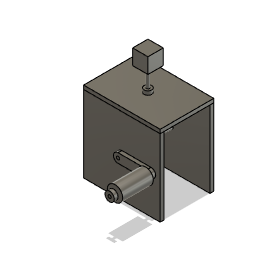
12. カム機構 (Autodesk Fusion 360 design; units mm, degrees)
description: Spur Gear; Module: 2.000000; Num Teeth: 18; Pressure Angle: 20.000000; Backlash: 0.00 mm
description: Spur Gear; Module: 2.000000; Num Teeth: 12; Pressure Angle: 20.000000; Backlash: 0.00 mm
Autodesk Fusion 360 part; units mm, degrees
sketch "スケッチ2" plane through (0, 0, 0) normal (0, 0, 1) x (1, 0, 0)
  line L0 (-25, 0) -> (25, 0)
  line L1 (25, 0) -> (25, 50)
  line L2 (25, 50) -> (-25, 50)
  line L3 (-25, 50) -> (-25, 0)
  circle A0 centre (0, 25) radius 1
  line L4 (3, 57) -> (22, 57)
  arc A1 (22, 57) -> (22, 63) centre (22, 60) ccw
  line L5 (22, 63) -> (3, 63)
  arc A2 (3, 63) -> (3, 57) centre (3, 60) ccw
  line L6 (0, 60) -> (25, 60) construction
  circle A3 centre (3, 60) radius 1
  circle A4 centre (22, 60) radius 1
  circle A5 centre (-15, 60) radius 3
  circle A6 centre (-15, 60) radius 1
  circle A7 centre (-35, 60) radius 5
  circle A8 centre (-35, 60) radius 1.25
  dimension "d1" = 2
  dimension "d16" = 2
  dimension "d21" = 2.5
  constraint horizontal L0
  constraint vertical L1
  constraint horizontal L2
  constraint vertical L3
  constraint tangent L4 A1
  constraint tangent A1 L5
  constraint parallel L4 L5
  constraint tangent L5 A2
  constraint tangent L4 A2
  constraint midpoint A2 L6.start
  constraint midpoint A1 L6.end
  constraint horizontal L6
  constraint concentric A2 A3
  constraint concentric A1 A4
  constraint concentric A5 A6
  constraint concentric A7 A8
  measures "d1" diameter of A0
  measures "d16" diameter of A3
  measures "d21" diameter of A8
extrude "押し出し1" add sketch "スケッチ2" along normal blind 2.5 contours L0 L1 L2 L3 makes body 1
cylinder "円柱プリミティブ1" add diameter 2 height 37.5 placed x (1, 0, 0) y (0, 1, 0) z (0, 0, 1) at (50, 0, 0) separate body makes body 2
extrude "押し出し2" add sketch "スケッチ2" along normal blind 2.5 separate body contours L4 A1 L5 A2 makes body 3
extrude "押し出し3" add sketch "スケッチ2" along normal blind 2.5 separate body contours A5 makes body 4
sketch "スケッチ5" plane through (0, 0, 0) normal (0, 1, 0) x (1, 0, 0)
extrude "押し出し4" add sketch "スケッチ2" along normal blind 20 separate body contours A7 makes body 5
cylinder "円柱プリミティブ2" add diameter 2 height 27 placed x (1, 0, 0) y (0, 1, 0) z (0, 0, 1) at (-25, 60, 0) separate body makes body 6
copy_body "ボディ -> コンポーネント1" bodies 1 removing the originals makes body 7 in component "土台"
copy_body "ボディ -> コンポーネント2" bodies 2 removing the originals makes body 8 in component "軸1"
copy_body "ボディ -> コンポーネント3" bodies 3 removing the originals makes body 9 in component "レバー"
copy_body "ボディ -> コンポーネント4" bodies 4 removing the originals makes body 10 in component "止め輪1"
copy_body "ボディ -> コンポーネント5" bodies 5 removing the originals makes body 11 in component "ハンドル"
copy_body "ボディ -> コンポーネント6" bodies 6 removing the originals makes body 12 in component "軸2"
sketch "スケッチ7" plane through (0, 0, 0) normal (0, 0, 1) x (1, 0, 0)
  line L0 (30, 15) -> (80, 15)
  line L1 (80, 15) -> (80, 50)
  line L2 (80, 50) -> (30, 50)
  line L3 (30, 50) -> (30, 15)
  circle A0 centre (55, 33) radius 1
  circle A1 centre (90, 0) radius 1
  circle A2 centre (100, 0) radius 2.5
  circle A3 centre (100, 0) radius 1
  constraint horizontal L0
  constraint vertical L1
  constraint horizontal L2
  constraint vertical L3
  constraint concentric A2 A3
extrude "押し出し1'" add sketch "スケッチ7" along normal blind 2.5 separate body contours L0 L1 L2 L3 makes body 13 in component "天板"
extrude "押し出し1''" add sketch "スケッチ7" along normal blind 30 separate body contours A1 makes body 14 in component "軸3"
extrude "押し出し1'''" add sketch "スケッチ7" along normal blind 2.5 separate body contours A2 makes body 15 in component "止め輪2"
box "直方体プリミティブ1" add length 10 width 10 height 10 placed x (0, -1, 0) y (1, 0, 0) z (0, 0, 1) at (90, 20, 0) separate body makes body 16 in component "キューブ"
cylinder "円柱プリミティブ1'" cut diameter 2 height -5 placed x (1, 0, 0) y (0, 1, 0) z (0, 0, 1) at (95, 15, 10) bodies 16 in component "キューブ"
extrude "押し出し1''''" add sketch "スケッチ7" along normal blind 2.5 separate body contours A2 makes body 17 in component "止め輪2 (1)"
copy_body "ボディのコピーと貼り付け1" bodies 7 makes body 18 in component "土台"
move_body "移動1" bodies 18 to x (1, 0, 0) y (0, 1, 0) z (0, 0, 1) at (0, 0, -32.5) in component "土台"
component "止め輪1" placed x (1, 0, 0) y (0, 1, 0) z (0, 0, 1) at (15, -35, -2.5)
component "止め輪2 (1)" placed x (1, 0, 0) y (0, 0, 1) z (0, -1, 0) at (-100, 55, -14.5)
component "底面" placed x (1, 0, 0) y (0, 1, 0) z (0, 0, 1) at (0, 0, 0)
component "原動節" placed x (1, 0, 0) y (0, 1, 0) z (0, 0, 1) at (0, 0, 0)
component "従動節" placed x (1, 0, 0) y (0, 1, 0) z (0, 0, 1) at (0, 0, 0)
component "筐体" placed x (1, 0, 0) y (0, 1, 0) z (0, 0, 1) at (0, 0, 0)
component "軸1" placed x (1, 0, 0) y (0, 1, 0) z (0, 0, 1) at (-50, 25, -32.5) in component "原動節"
component "レバー" placed x (1, 0, 0) y (0, 1, 0) z (0, 0, 1) at (-3, -35, 2.5) in component "原動節"
component "止め輪1" placed x (1, 0, 0) y (0, 1, 0) z (0, 0, 1) at (34, -35, 27) in component "原動節"
component "軸2" placed x (1, 0, 0) y (0, 1, 0) z (0, 0, 1) at (44, -35, 2.5) in component "原動節"
component "ハンドル" placed x (1, 0, 0) y (0, 1, 0) z (0, 0, 1) at (54, -35, 6) in component "原動節"
component "Spur Gear (18 teeth)" placed x (1, 0, 0) y (0, 1, 0) z (0, 0, 1) at (0, 0, 0) in component "原動節"
component "キューブ" placed x (-1, 0, 0) y (0, 0, -1) z (0, -1, 0) at (95, 77.5, 0.5) in component "従動節"
component "Spur Gear (12 teeth)" placed x (-1, 0, 0) y (0, 0, 1) z (0, 1, 0) at (0, 42.5, -14.5) in component "従動節"
component "止め輪2" placed x (1, 0, 0) y (0, 0, 1) z (0, -1, 0) at (-100, 55, -14.5) in component "従動節"
component "軸3" placed x (-1, 0, 0) y (0, 0, 1) z (0, 1, 0) at (90, 42.5, -14.5) in component "従動節"
component "土台" placed x (1, 0, 0) y (0, 1, 0) z (0, 0, 1) at (0, 0, 0) in component "筐体"
component "天板" placed x (1, 0, 0) y (0, 0, 1) z (0, -1, 0) at (-55, 52.5, -47.5) in component "筐体"
named bodies: "軸1"
